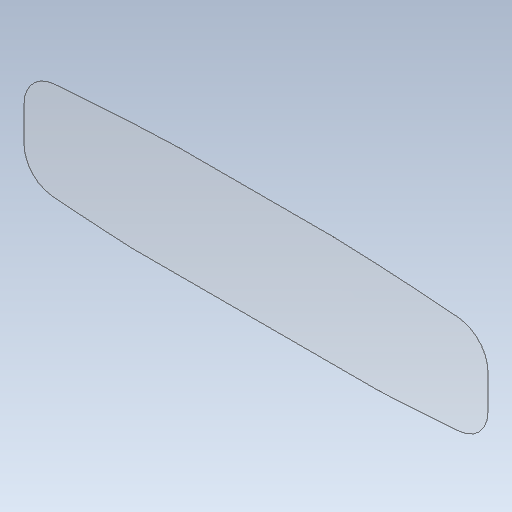
# Autodesk Inventor part: 7 Segment Clock Blanking Plate
Saved by Autodesk Inventor 2021 (Build 250183000, 183)
## iProperties
Created: 2020-06-27
Part Number: 7 Segment Clock Blanking Plate
Material: PMMA Plastic
Document SubType Name: Modeling
Designer: dech3
Density: 1.188 g/cm^3
Appearance: Polycarbonate - Clear
Author: dech3
Autodesk Inventor part; units mm, degrees
ref_plane "YZ Plane" through (0, 0, 0) normal (1, 0, 0) x (0, 1, 0)
ref_plane "XZ Plane" through (0, 0, 0) normal (0, 1, 0) x (-1, 0, 0)
ref_plane "XY Plane" through (0, 0, 0) normal (0, 0, 1) x (1, 0, 0)
sketch "Clock Front Face Outline" plane through (0, 0, 0) normal (0, 0, 1) x (1, 0, 0)
  arc A0 (261.5609, 58.5131) -> (100.3256, 67.9894) centre (0, -3015.4231) ccw
  arc A1 (-100.3256, 67.9894) -> (-261.5609, 58.5131) centre (0, -3015.4231) ccw
  line L0 (-159.5034, -75) -> (159.5034, -75)
  arc A2 (-263.2612, -68.2167) -> (-160.4975, -74.9753) centre (0, 3150) ccw
  arc A3 (160.4975, -74.9753) -> (263.2612, -68.2167) centre (0, 3150) ccw
  arc A4 (300, 16.6643) -> (261.5609, 58.5131) centre (258, 16.6643) ccw
  arc A5 (263.2612, -68.2167) -> (300, -28.3498) centre (260, -28.3498) ccw
  arc A6 (-300, -28.3498) -> (-263.2612, -68.2167) centre (-260, -28.3498) ccw
  arc A7 (-261.5609, 58.5131) -> (-300, 16.6643) centre (-258, 16.6643) ccw
  arc A8 (-99.6752, 68) -> (-100.3256, 67.9894) centre (-99.6752, 48) ccw
  arc A9 (100.3256, 67.9894) -> (99.6752, 68) centre (99.6752, 48) ccw
  arc A10 (159.5034, -75) -> (160.4975, -74.9753) centre (159.5034, -55) ccw
  arc A11 (-160.4975, -74.9753) -> (-159.5034, -75) centre (-159.5034, -55) ccw
  line L1 (-99.6752, 68) -> (99.6752, 68)
  line L2 (300, 16.6643) -> (300, -28.3498)
  line L3 (-300, -28.3498) -> (-300, 16.6643)
  point P0 (0, -2.2582)
  point P1 (-300, 55)
  point P2 (300, 55)
  point P3 (-300, -65)
  point P4 (300, -65)
  point P5 (-160, -75)
  point P6 (160, -75)
  point P7 (-100, 68)
  point P8 (100, 68)
  dimension "d0" = 600
  dimension "d1" = 120
  dimension "d2" = 120
  dimension "d3" = 140
  dimension "d4" = 140
  dimension "d5" = 200
  dimension "d6" = 200
  dimension "d7" = 200
  dimension "d8" = 320
  dimension "d9" = 143
  dimension "d10" = 10
  dimension "d11" = 10
  dimension "d12" = 13
  dimension "d13" = 13
  dimension "d14" = 42
  dimension "d15" = 40
  dimension "d16" = 40
  dimension "d17" = 42
  dimension "d18" = 20
  measures "d0" distance between parallel lines of L2 L3
  measures "d1" distance of point (-300, 55) point (-300, -65)
  measures "d2" distance of point (300, 55) point (300, -65)
  measures "d3" horizontal distance of point (-300, -65) point (-160, -75)
  measures "d4" horizontal distance of point (300, -65) point (160, -75)
  measures "d5" horizontal distance of point (-300, 55) point (-100, 68)
  measures "d6" horizontal distance of point (300, 55) point (100, 68)
  measures "d7" distance of point (100, 68) point (-100, 68)
  measures "d8" distance of point (160, -75) point (-160, -75)
  measures "d9" distance from line of L0 point (-100, 68)
  measures "d10" vertical distance of point (-300, -65) point (-160, -75)
  measures "d11" vertical distance of point (300, -65) point (160, -75)
  measures "d12" vertical distance of point (100, 68) point (300, 55)
  measures "d13" vertical distance of point (-100, 68) point (-300, 55)
  measures "d14" radius of A4
  measures "d15" radius of A5
  measures "d16" radius of A6
  measures "d17" radius of A7
  measures "d18" radius of A8
sketch "Sketch1" plane through (0, 0, 0) normal (0, 0, 1) x (1, 0, 0)
  arc A0 (261.5609, 58.5131) -> (100.3256, 67.9894) centre (0, -3015.4231) ccw
  arc A1 (-100.3256, 67.9894) -> (-261.5609, 58.5131) centre (0, -3015.4231) ccw
  line L0 (-159.5034, -75) -> (159.5034, -75)
  arc A2 (-263.2612, -68.2167) -> (-160.4975, -74.9753) centre (0, 3150) ccw
  arc A3 (160.4975, -74.9753) -> (263.2612, -68.2167) centre (0, 3150) ccw
  arc A4 (300, 16.6643) -> (261.5609, 58.5131) centre (258, 16.6643) ccw
  arc A5 (263.2612, -68.2167) -> (300, -28.3498) centre (260, -28.3498) ccw
  arc A6 (-300, -28.3498) -> (-263.2612, -68.2167) centre (-260, -28.3498) ccw
  arc A7 (-261.5609, 58.5131) -> (-300, 16.6643) centre (-258, 16.6643) ccw
  arc A8 (-99.6752, 68) -> (-100.3256, 67.9894) centre (-99.6752, 48) ccw
  arc A9 (100.3256, 67.9894) -> (99.6752, 68) centre (99.6752, 48) ccw
  arc A10 (159.5034, -75) -> (160.4975, -74.9753) centre (159.5034, -55) ccw
  arc A11 (-160.4975, -74.9753) -> (-159.5034, -75) centre (-159.5034, -55) ccw
  line L1 (-99.6752, 68) -> (99.6752, 68)
  line L2 (300, 16.6643) -> (300, -28.3498)
  line L3 (-300, -28.3498) -> (-300, 16.6643)
  point P0 (0, 0)
  point P1 (0, 0)
  dimension "d19" = 300
  dimension "d20" = 75
extrude "Extrusion1" add sketch "Sketch1" along normal blind 0.5
body "Solid1"
